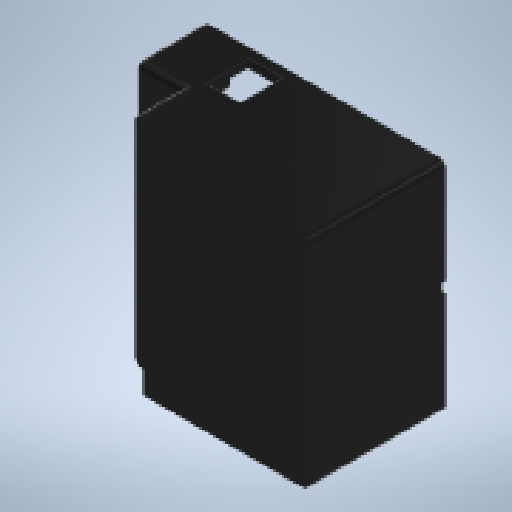
# Autodesk Inventor part: ND.ForagingFeeder.ApplicationBoard.Enclosure.Bottom
Saved by Autodesk Inventor 2023.2 (Build 272271000, 271)
## iProperties
Created: 2022-05-17
Part Number: ND.ForagingFeeder.ApplicationBoard.Enclosure.Bottom
Material: Generic
Document SubType Name: Modeling
Designer: Graeme
Density: 1 g/cm^3
Appearance: Default
Author: Graeme
Autodesk Inventor part; units mm, degrees
ref_plane "YZ Plane" through (0, 0, 0) normal (1, 0, 0) x (0, 1, 0)
ref_plane "XZ Plane" through (0, 0, 0) normal (0, 1, 0) x (-1, 0, 0)
sketch "Sketch1" plane through (0, 0, 0) normal (0, 1, 0) x (0, 0, -1)
  line L0 (6, 21.8796) -> (6, -21.8796) construction
  line L1 (12, 21.2597) -> (12, -21.2597) construction
  line L2 (18, 21.4434) -> (18, -21.4434) construction
  line L3 (0, 46.8587) -> (0, -46.8587) construction
  line L4 (0, 0) -> (37.1605, 0) construction
  line L5 (6, -8.1) -> (0, -8.1) construction
  line L6 (18, 8) -> (0, 8) construction
  line L7 (0, 12) -> (47.1795, 12) construction
  line L8 (35, 21.4434) -> (35, -52.3352) construction
  line L9 (35, -15) -> (0, -15) construction
  line L10 (55, 19.9798) -> (55, -19.9152) construction
  line L11 (53, -52) -> (0, -52) construction
  line L12 (35, 12) -> (18, 12)
  line L13 (18, 0) -> (6.2, 0)
  line L14 (6.2, -8.3) -> (6.2, 0)
  line L15 (6.2, -8.3) -> (0.2, -8.3)
  line L16 (0.2, -8.3) -> (0.2, -52)
  line L17 (18, 0) -> (18, 12)
  line L18 (2.2, -50) -> (2.2, -10.3)
  line L19 (2.2, -10.3) -> (8.2, -10.3)
  line L20 (8.2, -10.3) -> (8.2, -2)
  line L21 (8.2, -2) -> (20, -2)
  line L22 (20, -2) -> (20, 10)
  line L23 (20, 10) -> (35, 10)
  line L24 (35, 10) -> (35, 12)
  line L25 (0.2, -52) -> (35, -52)
  line L26 (35, -52) -> (35, -50)
  line L27 (35, -50) -> (2.2, -50)
  point P0 (6, 0)
  point P1 (12, 0)
  point P2 (35, -51)
  point P3 (35, 11)
  dimension "d0" = 6
  dimension "d1" = 6
  dimension "d2" = 6
  dimension "d3" = 8.1
  dimension "d4" = 8
  dimension "d5" = 4
  dimension "d6" = 35
  dimension "d7" = 27
  dimension "d8" = 20
  dimension "d9" = 64
  dimension "d10" = 0.2
  dimension "d11" = 0.2
  dimension "d12" = 0.2
  dimension "d13" = 2
  dimension "d26" = 2
  dimension "d27" = 2
  constraints: 56 end point, 17 point on line, 8 perpendicular, 7 vertical, 6 midpoint, 2 collinear, 2 horizontal, 1 coincident, 1 vertical alignment, 4 other
  measures "d0" distance between parallel lines of L3 L0
  measures "d1" distance between parallel lines of L0 L1
  measures "d2" distance between parallel lines of L1 L2
  measures "d3" distance between parallel lines of L5 L4
  measures "d4" distance between parallel lines of L6 L4
  measures "d5" distance between parallel lines of L7 L6
  measures "d6" distance between parallel lines of L3 L8
  measures "d7" distance between parallel lines of L9 L7
  measures "d8" distance between parallel lines of L10 L8
  measures "d9" distance between parallel lines of L11 L7
  measures "d10" distance between parallel lines of L3 L16
  measures "d11" distance between parallel lines of L5 L15
  measures "d12" distance between parallel lines of L0 L14
  measures "d13" distance between parallel lines of L16 L18
  measures "d26" distance of L25.end L26.end
  measures "d27" distance between parallel lines of L15 L19
extrude "Extrusion1" add sketch "Sketch1" along normal mid plane 57.325
sketch "Sketch2" plane through (2, -28.6625, -20) normal (1, 0, 0) x (0, 0, -1)
  line L0 (-27, 28.6625) -> (22, 28.6625) projected
  line L1 (-2, 0) -> (-2, 57.325) projected
  line L2 (-8, 48.5905) -> (-8, 8.7345) construction
  point P0 (-20, 28.6625)
  point P1 (-8, 28.6625)
  point P2 (-8, 46.1625)
  point P3 (-8, 11.1625)
  dimension "d16" = 17.5
  dimension "d17" = 17.5
  dimension "d18" = 6
  constraints: 3 point on line, 2 end point, 1 midpoint, 1 vertical
  measures "d16" distance from line of L0 point (-8, 46.163)
  measures "d17" distance of point (-8, 28.663) point (-8, 11.162)
  measures "d18" distance between parallel lines of L2 L1
hole "Hole1" at (2, 17.5, -12) at (2, -17.5, -12) direction (-1, 0, 0) diameter 3.2 depth 4
sketch "Sketch3" plane through (52, -28.6625, -35) normal (1, 0, 0) x (0, 0, -1)
  line L0 (0, 0) -> (0, 57.325) projected
  line L1 (0, 0) -> (-34.8, 0)
  line L2 (-34.8, 0) -> (-34.8, 2)
  line L3 (-34.8, 2) -> (0, 2)
  line L4 (0, 2) -> (0, 0)
  line L5 (0, 57.325) -> (-32.8, 57.325) projected
  line L6 (-34.8, 57.325) -> (-34.8, 0) projected
  line L7 (0, 57.325) -> (-34.8, 57.325)
  line L8 (-34.8, 57.325) -> (-34.8, 55.325)
  line L9 (-34.8, 55.325) -> (0, 55.325)
  line L10 (0, 55.325) -> (0, 57.325)
  point P0 (-35, 28.6625)
  point P1 (-32.8, 57.325)
  point P2 (0, 2)
  dimension "d28" = 2
  dimension "d29" = 2
  constraints: 16 end point, 4 parallel, 2 horizontal, 2 perpendicular, 2 point on line
  measures "d28" distance of L1.end L2.end
  measures "d29" distance of L8.end L7.end
extrude "Extrusion2" add sketch "Sketch3" against normal up to next contours L1 L2 L3 L0 | L9 L6 L7 L5 L0
ref_plane "Work Plane1" through (52, -28.6625, -33.4) normal (0, 0, -1) x (-1, 0, 0)
sketch "Sketch4" plane through (52, -28.6625, -33.4) normal (0, 0, -1) x (-1, 0, 0)
  line L0 (62, 2) -> (62, 55.325) projected
  line L1 (62, 55.325) -> (54, 55.325)
  line L2 (54, 55.325) -> (54, 47.325)
  line L3 (54, 47.325) -> (62, 47.325)
  line L4 (62, 47.325) -> (62, 55.325)
  line L5 (2, 2) -> (62, 2) projected
  line L6 (62, 2) -> (54, 2)
  line L7 (54, 2) -> (54, 10)
  line L8 (54, 10) -> (62, 10)
  line L9 (62, 10) -> (62, 2)
  line L10 (2, 2) -> (2, 55.325) projected
  line L11 (2, 2) -> (10, 2)
  line L12 (10, 2) -> (10, 10)
  line L13 (10, 10) -> (2, 10)
  line L14 (2, 10) -> (2, 2)
  line L15 (2, 55.325) -> (10, 55.325)
  line L16 (10, 55.325) -> (10, 47.325)
  line L17 (10, 47.325) -> (2, 47.325)
  line L18 (2, 47.325) -> (2, 55.325)
  point P0 (52, 28.6625)
  point P1 (2, 47.325)
  point P2 (2, 10)
  point P3 (10, 2)
  point P4 (54, 2)
  point P5 (62, 47.325)
  dimension "d33" = 8
  dimension "d34" = 8
  dimension "d35" = 8
  dimension "d36" = 8
  dimension "d37" = 8
  dimension "d38" = 8
  dimension "d39" = 8
  dimension "d40" = 8
  constraints: 32 end point, 8 parallel, 4 horizontal, 4 perpendicular
  measures "d33" distance of L3.end L2.end
  measures "d34" distance of L2.end L1.end
  measures "d35" distance of L7.end L8.end
  measures "d36" distance of L6.end L7.end
  measures "d37" distance of L13.end L12.end
  measures "d38" distance of L12.end L11.end
  measures "d39" distance of L16.end L17.end
  measures "d40" distance of L15.end L16.end
extrude "Extrusion3" add sketch "Sketch4" against normal up to next
fillet "Fillet1" radius 2 12 edges at (-10, 18.6625, -26.7) (-2, 18.6625, -26.7) (-2, 26.6625, -26.7) (-10, -18.6625, -26.7) (-2, -18.6625, -26.7) (-2, -26.6625, -26.7) (42, -26.6625, -17.8) (42, -18.6625, -17.8) (50, -18.6625, -17.8) (50, 18.6625, -17.8) (42, 18.6625, -17.8) (42, 26.6625, -17.8)
sketch "Sketch5" plane through (52, -28.6625, -33.4) normal (0, 0, -1) x (-1, 0, 0)
  circle A0 centre (57, 7) radius 1.6 projected
  circle A1 centre (7, 7.325) radius 1.6 projected
  circle A2 centre (7, 50.325) radius 1.6 projected
  circle A3 centre (57, 50.325) radius 1.6 projected
  point P0 (52, 28.6625)
  constraints: 4 coincident
hole "Hole2" at (-5, 21.6625, -33.4) at (45, 21.6625, -33.4) at (45, -21.3375, -33.4) at (-5, -21.6625, -33.4) direction (0, 0, 1) diameter 2.459 depth 10 thread size "M3x0.5" class "6H" standard "ISO Metric profile"
fillet "Fillet2" radius 2 4 edges at (-12, -28.6625, -26.5) (-12, 28.6625, -26.5) (52, 28.6625, -17.6) (52, -28.6625, -17.6)
fillet "Fillet3" radius 1 4 edges at (-10, -26.6625, -34.2) (50, -26.6625, -34.2) (50, 26.6625, -34.2) (-10, 26.6625, -34.2)
sketch "Sketch6" plane through (2, -26.6625, -8.2) normal (1, 0, 0) x (0, 0, -1)
  line L0 (11.8, 53.325) -> (0, 53.325) projected
  line L1 (11.8, 53.325) -> (0, 53.325)
  line L2 (0, 53.325) -> (0, 0)
  line L3 (0, 0) -> (11.8, 0)
  line L4 (11.8, 0) -> (11.8, 53.325)
  circle A0 centre (3.8, 44.1625) radius 1.6 projected
  circle A1 centre (3.8, 44.1625) radius 1.6 projected
  circle A2 centre (3.8, 9.1625) radius 1.6 projected
  point P0 (-8.2, 26.6625)
  constraints: 8 end point, 2 parallel, 1 horizontal, 1 perpendicular
extrude "Extrusion4" add sketch "Sketch6" along normal blind 1
sketch "Sketch7" plane through (3, -26.6625, -8.2) normal (1, 0, 0) x (0, 0, -1)
  circle A0 centre (3.8, 44.1625) radius 1.6 projected
  circle A1 centre (3.8, 44.1625) radius 4.6
  circle A2 centre (3.8, 9.1625) radius 1.6 projected
  circle A3 centre (3.8, 9.1625) radius 4.6
  line L0 (0, 0) -> (0, 53.325) projected
  line L1 (3.8, 48.7625) -> (0, 48.7625)
  line L2 (3.8, 39.5625) -> (0, 39.5625)
  line L3 (3.8, 13.7625) -> (0, 13.7625)
  line L4 (3.8, 4.5625) -> (0, 4.5625)
  point P0 (-8.2, 26.6625)
  dimension "d55" = 9.2
  dimension "d56" = 9.2
  constraints: 8 end point, 4 coincident, 4 perpendicular, 4 point on circle, 4 point on line, 4 tangent, 2 centre point
  measures "d55" diameter of A1
  measures "d56" diameter of A3
extrude "Extrusion5" add sketch "Sketch7" along normal blind 2 contours A1 L0 | A1 L0 L1 | L2 L0 A1 | A3 L0 | A3 L0 L3 | L4 L0 A3 picked at (0.7333, 44.1625) picked at (0.7333, 9.1625)
sketch "Sketch14" plane through (5, -26.6625, -8.2) normal (1, 0, 0) x (0, 0, -1)
  circle A0 centre (3.8, 44.1625) radius 4.6
  circle A1 centre (3.8, 9.1625) radius 4.6
  circle A2 centre (3.8, 44.1625) radius 1.6 projected
  circle A3 centre (3.8, 9.1625) radius 1.6 projected
  point P0 (-8.2, 26.6625)
  dimension "d87" = 9.2
  dimension "d88" = 9.2
  constraints: 2 centre point, 2 concentric
  measures "d87" diameter of A0
  measures "d88" diameter of A1
extrude "Extrusion10" cut sketch "Sketch14" along normal up to surface (5.3 mm away)
sketch "Sketch8" plane through (5, -26.6625, -8.2) normal (1, 0, 0) x (0, 0, -1)
  circle A0 centre (3.8, 44.1625) radius 1.6 projected
  circle A1 centre (3.8, 9.1625) radius 1.6 projected
  point P0 (-8.2, 26.6625)
  constraints: 2 coincident
hole "Hole3" at (5, 17.5, -12) at (5, -17.5, -12) direction (-1, 0, 0) diameter 4.5 depth 10 countersink diameter 9.2 countersink angle 90 clearance for "Countersunk Flat Head Hex Socket Screw ISO 10642" size "M4" standard "ISO"
fillet "Fillet4" radius 1 43 edges at (3, 24.3812, -8.2) (3, 17.5, -16.6) (3, 12.9, -10.1) (3, 22.1, -10.1) (3, 0, -8.2) (3, -22.1, -10.1) (3, -12.9, -10.1) (3, -17.5, -16.6) (3, -24.3813, -8.2) (3, 0, -20) (10.3, 0, -2.2) (41.4142, 26.0767, -2.2) (42, 22.6625, -2.2) (42.5858, 19.2483, -2.2) (46, 18.6625, -2.2) (49.4142, 18.0767, -2.2) (50, 0, -2.2) (49.4142, -18.0767, -2.2) (46, -18.6625, -2.2) (42.5858, -19.2483, -2.2) (42, -22.6625, -2.2) (41.4142, -26.0767, -2.2) (25.15, -26.6625, -2.2) (25.15, 26.6625, -2.2) (-9.4142, 18.0767, -20) (-6, 18.6625, -20) (-2.5858, 19.2483, -20) (-2, 22.6625, -20) (-1.4142, 26.0767, -20) (1.5, 26.6625, -20) (-9.4142, -18.0767, -20) (-6, -18.6625, -20) (-2.5858, -19.2483, -20) (-2, -22.6625, -20) (-1.4142, -26.0767, -20) (1.5, -26.6625, -20) (-10, 0, -20) (6.65, 26.6625, -8.2) (3, 26.6625, -14.1) (10.3, 26.6625, -5.2) (3, -26.6625, -14.1) (6.65, -26.6625, -8.2) (10.3, -26.6625, -5.2)
sketch "Sketch9" plane through (50, -28.6625, -35) normal (0, 0, -1) x (-1, 0, 0)
  arc A0 (-2, 2) -> (0, 0) centre (0, 2) ccw projected
  line L0 (60, 0) -> (0, 0) projected
  arc A1 (60, 0) -> (62, 2) centre (60, 2) ccw projected
  line L1 (62, 2) -> (62, 55.325) projected
  arc A2 (62, 55.325) -> (60, 57.325) centre (60, 55.325) ccw projected
  line L2 (0, 57.325) -> (60, 57.325) projected
  arc A3 (0, 57.325) -> (-2, 55.325) centre (0, 55.325) ccw projected
  line L3 (-2, 2) -> (-2, 55.325) projected
  line L4 (1, 55.325) -> (59, 55.325) projected
  arc A4 (60, 54.325) -> (59, 55.325) centre (59, 54.325) ccw projected
  line L5 (60, 3) -> (60, 54.325) projected
  arc A5 (59, 2) -> (60, 3) centre (59, 3) ccw projected
  line L6 (1, 2) -> (59, 2) projected
  arc A6 (0, 3) -> (1, 2) centre (1, 3) ccw projected
  line L7 (0, 3) -> (0, 54.325) projected
  arc A7 (1, 55.325) -> (0, 54.325) centre (1, 54.325) ccw projected
  line L8 (61, 55.325) -> (61, 2)
  arc A8 (60, 1) -> (61, 2) centre (60, 2) ccw
  line L9 (60, 1) -> (0, 1)
  arc A9 (-1, 2) -> (0, 1) centre (0, 2) ccw
  line L10 (-1, 2) -> (-1, 55.325)
  arc A10 (0, 56.325) -> (-1, 55.325) centre (0, 55.325) ccw
  line L11 (0, 56.325) -> (60, 56.325)
  arc A11 (61, 55.325) -> (60, 56.325) centre (60, 55.325) ccw
  point P0 (50, 28.6625)
  dimension "d67" = 1
  constraints: 8 end point, 8 point on circle, 4 centre point, 7 other
  measures "d67" distance between parallel lines of L1 L8
extrude "Extrusion6" add sketch "Sketch9" along normal blind 1 contours L3 A3 L2 A2 L1 A1 L0 A0
fillet "Fillet5" radius 2 7 edges at (-11.4142, 28.0767, -18) (-12, 0, -18) (-11.4142, -28.0767, -18) (-5, -28.6625, -18) (-5, 28.6625, -18) (0, 28.6625, -12.1) (0, -28.6625, -12.1)
sketch "Sketch10" plane through (0, -28.6625, 0) normal (0, -1, 0) x (1, 0, 0)
  line L0 (49, -35) -> (-9, -35) projected
  line L1 (49, -35) -> (-9, -35) projected
  line L2 (36.645, -36) -> (20.905, -36)
  line L3 (20.905, -36) -> (20.905, -35)
  line L4 (20.905, -35) -> (36.645, -35)
  line L5 (36.645, -35) -> (36.645, -36)
  line L6 (50, -35) -> (-10, -35) projected
  line L7 (14.625, -36) -> (7.375, -36)
  line L8 (7.375, -36) -> (7.375, -35)
  line L9 (7.375, -35) -> (14.625, -35)
  line L10 (14.625, -35) -> (14.625, -36)
  line L11 (20.905, -44.491) -> (20.905, -36) projected
  line L12 (14.625, -36) -> (14.625, -38.62) projected
  line L13 (7.375, -38.62) -> (7.375, -36) projected
  line L14 (36.645, -36) -> (36.645, -44.491) projected
  point P0 (0, 0)
  constraints: 16 end point, 4 parallel, 2 horizontal, 2 perpendicular, 2 point on line, 1 other
extrude "Extrusion7" cut sketch "Sketch10" against normal blind 2
sketch "Sketch11" plane through (0, 28.6625, 0) normal (0, 1, 0) x (1, 0, 0)
  line L0 (5.35, 33.0782) -> (8.55, 33.0782) projected
  line L1 (2.85, 33.0782) -> (5.35, 33.0782) projected
  line L2 (2.85, 22.8782) -> (2.85, 33.0782) projected
  line L3 (11.05, 22.8782) -> (2.85, 22.8782) projected
  line L4 (11.05, 33.0782) -> (11.05, 22.8782) projected
  line L5 (8.55, 33.0782) -> (11.05, 33.0782) projected
  circle A0 centre (6.95, 26.9782) radius 3.2 projected
  point P0 (0, 0)
extrude "Extrusion8" cut sketch "Sketch11" against normal blind 2 contours L0 L5 L4 L3 L2 L1 | A0
fillet "Fillet6" radius 1 10 edges at (2.85, 28.6625, -27.9782) (6.95, 28.6625, -33.0782) (11.05, 28.6625, -27.9782) (6.95, 28.6625, -22.8782) (36.645, -28.6625, -35.5) (28.775, -28.6625, -35) (20.905, -28.6625, -35.5) (14.625, -28.6625, -35.5) (11, -28.6625, -35) (7.375, -28.6625, -35.5)
sketch "Sketch13" plane through (52, -26.6625, -0.2) normal (1, 0, 0) x (0, 0, -1)
  line L0 (36.8, 28.1625) -> (34.8, 28.1625)
  line L1 (34.8, 28.1625) -> (34.8, 25.1625)
  line L2 (34.8, 25.1625) -> (36.8, 25.1625)
  line L3 (36.8, 25.1625) -> (36.8, 28.1625)
  line L4 (35.8, 53.325) -> (35.8, 0) projected
  line L5 (36.8, 28.1625) -> (34.8, 25.1625) construction
  line L6 (34.8, 28.1625) -> (36.8, 25.1625) construction
  point P0 (-0.2, 26.6625)
  point P1 (35.8, 26.6625)
  dimension "d83" = 2
  dimension "d84" = 3
  constraints: 12 end point, 3 midpoint, 2 parallel, 1 horizontal, 1 perpendicular
  measures "d83" distance of L2.end L1.end
  measures "d84" distance of L1.end L0.end
extrude "Extrusion9" cut sketch "Sketch13" against normal blind 3
equation "\"d10\" = Clearance"
equation "\"d11\" = Clearance"
equation "\"d12\" = Clearance"
equation "\"d27\" = d13"
equation "\"d17\" = d16"
equation "\"d67\" = LipWidth"
equation "\"d68\" = LipHeight"
equation "\"Clearance\" = 0.2"
equation "\"LipWidth\" = 1"
equation "\"LipHeight\" = 1"
body "Solid1"
